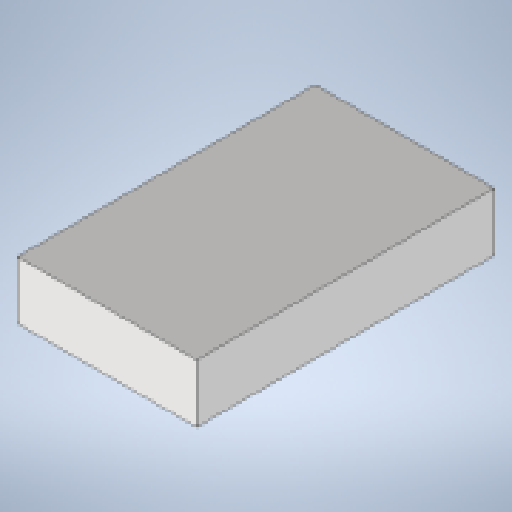
# Autodesk Inventor part: LiPo3000mAH
Saved by Autodesk Inventor 2025.1 (Build 291241000, 241)
## iProperties
Created: 2025-05-22
Part Number: LiPo3000mAH
Material: Generic
Document SubType Name: Modeling
Designer: User
Density: 1 g/cm^3
Appearance: Default
Author: User
Autodesk Inventor part; units mm, degrees
ref_plane "YZ Plane" through (0, 0, 0) normal (1, 0, 0) x (0, 1, 0)
ref_plane "XZ Plane" through (0, 0, 0) normal (0, 1, 0) x (-1, 0, 0)
ref_plane "XY Plane" through (0, 0, 0) normal (0, 0, 1) x (1, 0, 0)
sketch "Sketch1" plane through (0, 0, 0) normal (0, 0, 1) x (1, 0, 0)
  line L0 (-8.8755, 3.2604) -> (35.1245, 3.2604)
  line L1 (35.1245, 3.2604) -> (35.1245, -18.7396)
  line L2 (35.1245, -18.7396) -> (-8.8755, -18.7396)
  line L3 (-8.8755, -18.7396) -> (-8.8755, 3.2604)
  point P0 (0, 0)
  dimension "d0" = 44
  dimension "d1" = 22
  constraints: 8 end point, 2 parallel, 1 horizontal, 1 perpendicular
  measures "d0" distance of L1.end L2.end
  measures "d1" distance of L0.end L1.end
extrude "Extrusion1" add sketch "Sketch1" against normal blind 152
sketch "Sketch2" plane through (35.1245, -18.7396, 0) normal (1, 0, 0) x (0, 0, -1)
  line L0 (152, 22) -> (152, 0) projected
  line L1 (0, 22) -> (152, 22) projected
  line L2 (0, 0) -> (152, 0) projected
  line L3 (0, 0) -> (0, 22) projected
  point P0 (0, 18.7396)
extrude "Extrusion2" add sketch "Sketch2" along normal blind 20
sketch "Sketch3" plane through (-8.8755, -18.7396, -152) normal (0, -1, 0) x (1, 0, 0)
  line L0 (0, 152) -> (64, 152) projected
  line L1 (0, 0) -> (64, 0) projected
  line L2 (64, 0) -> (64, 152) projected
  line L3 (64, 0) -> (71, 0)
  line L4 (71, 0) -> (71, 152)
  line L5 (71, 152) -> (64, 152)
  line L6 (64, 152) -> (64, 0)
  point P0 (8.8755, 152)
  dimension "d6" = 64
  dimension "d7" = 7
  constraints: 8 end point, 2 parallel, 1 horizontal, 1 perpendicular
  measures "d6" distance of L0.start L0.end
  measures "d7" distance of L5.end L4.end
extrude "Extrusion3" add sketch "Sketch3" against normal up to surface (22 mm away)
sketch "Sketch4" plane through (-8.8755, -18.7396, -152) normal (0, -1, 0) x (1, 0, 0)
  line L0 (0, 152) -> (0, 0) projected
  line L1 (0, 152) -> (71, 152) projected
  line L2 (71, 0) -> (71, 152) projected
  line L3 (0, 152) -> (71, 152)
  line L4 (71, 152) -> (71, 34)
  line L5 (71, 34) -> (0, 34)
  line L6 (0, 34) -> (0, 152)
  point P0 (8.8755, 152)
  dimension "d10" = 152
  dimension "d11" = 118
  constraints: 8 end point, 2 parallel, 1 horizontal, 1 perpendicular, 1 point on line
  measures "d10" distance of L0.start L0.end
  measures "d11" distance of L3.end L4.end
extrude "Extrusion4" cut sketch "Sketch4" against normal blind 10 keep common part
sketch "Sketch5" plane through (0, 0, 0) normal (0, 0, 1) x (1, 0, 0)
  line L0 (62.1245, -18.7396) -> (62.1245, -8.7396) projected
  line L1 (-8.8755, -18.7396) -> (62.1245, -18.7396) projected
  line L2 (62.1245, -18.7396) -> (-8.8755, -18.7396)
  line L3 (-8.8755, -18.7396) -> (-8.8755, 4.2604)
  line L4 (-8.8755, 4.2604) -> (62.1245, 4.2604)
  line L5 (62.1245, 4.2604) -> (62.1245, -18.7396)
  line L6 (-8.8755, -8.7396) -> (62.1245, -8.7396) projected
  point P0 (0, 0)
  dimension "d14" = 10
  dimension "d15" = 23
  constraints: 8 end point, 2 parallel, 1 horizontal, 1 perpendicular
  measures "d14" distance of L0.start L0.end
  measures "d15" distance of L2.end L3.end
extrude "Extrusion5" add sketch "Sketch5" against normal up to surface (118 mm away) contours L6 L3 L4 L5
body "Solid1"
